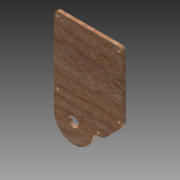
# Autodesk Inventor part: p1
Saved by Autodesk Inventor 2015 (Build 190159000, 159)
## iProperties
Created: 2016-02-03
Part Number: p1
Material: Generic
Document SubType Name: Modeling
Designer: david
Density: 1 g/cm^3
Appearance: Birch - Natural Polished
Author: david
Autodesk Inventor part; units mm, degrees
ref_plane "YZ Plane" through (0, 0, 0) normal (1, 0, 0) x (0, 1, 0)
ref_plane "XZ Plane" through (0, 0, 0) normal (0, 1, 0) x (-1, 0, 0)
ref_plane "XY Plane" through (0, 0, 0) normal (0, 0, 1) x (1, 0, 0)
sketch "Sketch1" plane through (0, 0, 0) normal (0, 1, 0) x (-1, 0, 0)
  line L0 (20, 45) -> (-20, 45)
  line L1 (-20, 45) -> (-20, -45)
  line L2 (-20, -45) -> (20, -45)
  line L3 (20, 45) -> (-20, -45) construction
  line L4 (-20, 45) -> (20, -45) construction
  arc A0 (-20, -45) -> (20, -45) centre (0, -45) ccw
  line L5 (20, 45) -> (20, -45)
  line L6 (-20, -45) -> (-50, -45)
  line L7 (-50, -45) -> (-50, 45)
  line L8 (-50, 45) -> (-20, 45)
  line L9 (-20, 45) -> (-20, -45)
  point P0 (0, 0)
  dimension "d0" = 40
  dimension "d1" = 90
  dimension "d26" = 30
  constraints: 20 end point, 3 midpoint, 3 parallel, 2 horizontal, 2 perpendicular, 2 point on circle, 1 centre point, 1 vertical
  measures "d0" distance of L2.end L1.end
  measures "d1" distance of L1.end L0.end
  measures "d26" distance of L7.end L8.end
extrude "Extrusion1" add sketch "Sketch1" along normal blind 3.6
sketch "Sketch2" plane through (0, 3.6, 0) normal (0, 1, 0) x (1, 0, 0)
  arc A0 (20, 45) -> (-20, 45) centre (0, 45) ccw projected
  circle A1 centre (0, 45) radius 5.15
  point P0 (0, 0)
  dimension "d4" = 10.3
  constraints: 1 centre point, 1 coincident
  measures "d4" diameter of A1
extrude "Extrusion2" cut sketch "Sketch2" against normal blind 3.6
fillet "Fillet1" radius 4 4 edges at (-20, 1.8, -45) (50, 1.8, 45) (-20, 1.8, 45) (20, 1.8, -45)
chamfer "Chamfer1" distance 20 angle 45 1 edges at (50, 1.8, -45)
fillet "Fillet2" radius 10 2 edges at (30, 1.8, -45) (50, 1.8, -25)
sketch "Sketch5" plane through (0, 0, 0) normal (0, -1, 0) x (1, 0, 0)
  circle A0 centre (25, -41.5) radius 1.625
  circle A1 centre (46.5, -21.5) radius 1.625
  circle A2 centre (46.5, 41.5) radius 1.625
  circle A3 centre (-16.5, -23.5) radius 1.625
  line L0 (25.8579, -45) -> (23.6643, -45) projected
  line L1 (50, 41) -> (50, -20.8579) projected
  line L2 (-20, -45) -> (-20, 41) projected
  line L3 (-16, 45) -> (46, 45) projected
  circle A4 centre (-16.5, 41.5) radius 1.625
  point P0 (0, 0)
  dimension "d31" = 3.25
  dimension "d32" = 3.25
  dimension "d34" = 3.25
  dimension "d35" = 3.25
  dimension "d36" = 3.5
  dimension "d37" = 3.5
  dimension "d38" = 3.5
  dimension "d40" = 25
  dimension "d41" = 20
  dimension "d42" = 3.5
  dimension "d43" = 3.5
  dimension "d48" = 3.25
  dimension "d49" = 3.5
  dimension "d50" = 3.5
  dimension "d52" = 65
  constraints: 5 centre point
  measures "d31" diameter of A0
  measures "d32" diameter of A1
  measures "d34" diameter of A2
  measures "d35" diameter of A3
  measures "d36" distance from line of L0 A0.centre
  measures "d37" distance from line of L1 A1.centre
  measures "d38" distance from line of L2 A3.centre
  measures "d40" distance from line of L1 A0.centre
  measures "d41" vertical distance of A1.centre A0.centre
  measures "d42" distance from line of A2.centre L3
  measures "d43" distance from line of L1 A2.centre
  measures "d48" diameter of A4
  measures "d49" distance from line of L3 A4.centre
  measures "d50" distance from line of L2 A4.centre
  measures "d52" distance of A4.centre A3.centre
extrude "Extrusion5" cut sketch "Sketch5" against normal blind 10
body "Solid1"
